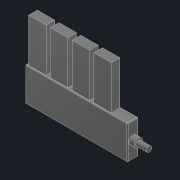
# Autodesk Inventor part: U3H-FC03BBK
Saved by Autodesk Inventor 2022 (Build 260153000, 153)
## iProperties
Created: 2021-08-30
Part Number: U3H-FC03BBK
Material: ABS プラスチック
Document SubType Name: Modeling
Designer: Yuta Kage
Density: 1.06 g/cm^3
Appearance: 滑らか - 黒
Author: Yuta Kage
Autodesk Inventor part; units mm, degrees
ref_plane "YZ Plane" through (0, 0, 0) normal (1, 0, 0) x (0, 1, 0)
ref_plane "XZ Plane" through (0, 0, 0) normal (0, 1, 0) x (-1, 0, 0)
ref_plane "XY Plane" through (0, 0, 0) normal (0, 0, 1) x (1, 0, 0)
sketch "スケッチ1" plane through (0, 0, 0) normal (0, 0, 1) x (1, 0, 0)
  line L0 (47, -15.5) -> (-47, -15.5)
  line L1 (-47, -15.5) -> (-47, 15.5)
  line L2 (-47, 15.5) -> (47, 15.5)
  line L3 (47, 15.5) -> (47, -15.5)
  line L4 (47, -15.5) -> (-47, 15.5) construction
  line L5 (-47, -15.5) -> (47, 15.5) construction
  point P0 (0, 0)
  dimension "d0" = 94
  dimension "d1" = 31
  constraints: 12 end point, 2 midpoint, 2 parallel, 1 horizontal, 1 perpendicular
  measures "d0" distance of L1.end L2.end
  measures "d1" distance of L2.end L0.start
extrude "押し出し1" add sketch "スケッチ1" along normal mid plane 10
sketch "スケッチ2" plane through (47, -15.5, 5) normal (1, 0, 0) x (0, 0, -1)
  circle A0 centre (5, 15.5) radius 4
  dimension "d4" = 8
  constraints: 1 centre point, 1 coincident
  measures "d4" diameter of A0
extrude "押し出し2" add sketch "スケッチ2" along normal blind 5
sketch "スケッチ3" plane through (52, 0, 0) normal (1, 0, 0) x (0, 0, -1)
  circle A0 centre (0, 0) radius 2.5
  dimension "d7" = 5
  constraints: 1 centre point, 1 coincident
  measures "d7" diameter of A0
extrude "押し出し3" add sketch "スケッチ3" along normal blind 10
fillet "フィレット1" radius 0.5 12 edges at (0, 15.5, 5) (47, 0, 5) (47, 15.5, 0) (47, -15.5, 0) (0, -15.5, 5) (0, 15.5, -5) (0, -15.5, -5) (47, 0, -5) (-47, 0, 5) (-47, 15.5, 0) (-47, 0, -5) (-47, -15.5, 0)
sketch "スケッチ4" plane through (-46.5, 15.5, -4.5) normal (0, 1, 0) x (1, 0, 0)
  line L0 (1.5, -0.5) -> (17.5, -0.5)
  line L1 (17.5, -0.5) -> (17.5, -8.5)
  line L2 (17.5, -8.5) -> (1.5, -8.5)
  line L3 (1.5, -8.5) -> (1.5, -0.5)
  line L4 (1.5, -0.5) -> (17.5, -8.5) construction
  line L5 (17.5, -0.5) -> (1.5, -8.5) construction
  line L6 (-0.5, 0) -> (-0.5, -9) projected
  point P0 (46.5, -4.5)
  point P1 (9.5, -4.5)
  point P2 (9.5, -4.5)
  dimension "d11" = 8
  dimension "d12" = 16
  dimension "d13" = 10
  constraints: 12 end point, 3 midpoint, 2 parallel, 1 horizontal, 1 horizontal alignment, 1 perpendicular
  measures "d11" distance of L0.end L1.end
  measures "d12" distance of L0.start L0.end
  measures "d13" distance from line of L6 point (9.5, -4.5)
extrude "押し出し4" add sketch "スケッチ4" along normal blind 40
pattern_linear "矩形状パターン1" count 4 spacing 20 along (1, 0, 0) of "押し出し4"
